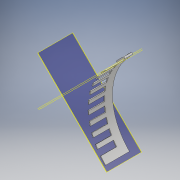
# Autodesk Inventor part: QuarterCircle
Saved by Autodesk Inventor 2018.3 (Build 223284000, 284)
## iProperties
Created: 2021-04-14
Part Number: QuarterCircle
Material: Generic
Document SubType Name: Modeling
Designer: swarmArena
Density: 1 g/cm^3
Appearance: Default
Author: swarmArena
Autodesk Inventor part; units mm, degrees
ref_plane "YZ Plane" through (0, 0, 0) normal (1, 0, 0) x (0, 1, 0)
ref_plane "XZ Plane" through (0, 0, 0) normal (0, 1, 0) x (-1, 0, 0)
ref_plane "XY Plane" through (0, 0, 0) normal (0, 0, 1) x (1, 0, 0)
sketch "Sketch1" plane through (0, 0, 0) normal (0, 1, 0) x (-1, 0, 0)
  circle A0 centre (0, 0) radius 111
  dimension "d13" = 222
  constraints: 1 centre point
  measures "d13" diameter of A0
extrude "Extrusion1" add sketch "Sketch1" along normal blind 45
sketch "Sketch2" plane through (0, 0, 0) normal (0, 1, 0) x (-1, 0, 0)
  circle A0 centre (0, 0) radius 109.5
  dimension "d16" = 219
  constraints: 1 centre point, 1 coincident
  measures "d16" diameter of A0
extrude "Extrusion2" cut sketch "Sketch2" along normal blind 50
sketch "Sketch3" plane through (0, 0, 0) normal (0, 1, 0) x (-1, 0, 0)
  line L0 (0, 0) -> (106.066, 106.066)
  line L1 (106.066, 106.066) -> (0, 212.132)
  line L2 (0, 212.132) -> (-106.066, 106.066)
  line L3 (-106.066, 106.066) -> (0, 0)
  line L4 (0, 0) -> (-106.066, -106.066)
  line L5 (-106.066, -106.066) -> (-212.132, 0)
  line L6 (-212.132, 0) -> (-106.066, 106.066)
  line L7 (-106.066, 106.066) -> (0, 0)
  line L8 (0, 0) -> (-106.066, -106.066)
  line L9 (-106.066, -106.066) -> (0, -212.132)
  line L10 (0, -212.132) -> (106.066, -106.066)
  line L11 (106.066, -106.066) -> (0, 0)
  dimension "d19" = 150
  dimension "d20" = 150
  dimension "d21" = 150
  dimension "d22" = 150
  dimension "d23" = 150
  dimension "d24" = 150
  constraints: 24 end point, 6 parallel, 3 perpendicular
  measures "d19" distance of L2.end L1.end
  measures "d20" distance of L1.end L0.end
  measures "d21" distance of L5.end L6.end
  measures "d22" distance of L4.end L5.end
  measures "d23" distance of L10.end L9.end
  measures "d24" distance of L9.end L8.end
extrude "Extrusion3" cut sketch "Sketch3" along normal blind 60
sketch "Sketch4" plane through (0, 0, 0) normal (1, 0, 0) x (0, 1, 0)
  line L0 (0, -77.4282) -> (0, 77.4282) projected
  line L1 (0, -4) -> (30, -4)
  line L2 (30, -4) -> (30, 6)
  line L3 (30, 6) -> (0, 6)
  line L4 (0, 6) -> (0, -4)
  line L5 (-32.9413, -3) -> (-32.9413, -15.7313) construction
  line L6 (-32.9413, -20) -> (-32.9413, -32.7313) construction
  line L7 (0, -21) -> (30, -21)
  line L8 (30, -11) -> (0, -11)
  line L9 (30, -21) -> (30, -11)
  line L10 (0, -11) -> (0, -21)
  line L11 (-32.9413, -37) -> (-32.9413, -49.7313) construction
  line L12 (0, -38) -> (30, -38)
  line L13 (30, -28) -> (0, -28)
  line L14 (30, -38) -> (30, -28)
  line L15 (0, -28) -> (0, -38)
  line L16 (-32.9413, -54) -> (-32.9413, -66.7313) construction
  line L17 (0, -55) -> (30, -55)
  line L18 (30, -45) -> (0, -45)
  line L19 (30, -55) -> (30, -45)
  line L20 (0, -45) -> (0, -55)
  line L21 (-32.9413, -71) -> (-32.9413, -83.7313) construction
  line L22 (0, -72) -> (30, -72)
  line L23 (30, -62) -> (0, -62)
  line L24 (30, -72) -> (30, -62)
  line L25 (0, -62) -> (0, -72)
  line L26 (0, 23) -> (0, 13)
  line L27 (0, 13) -> (30, 13)
  line L28 (30, 23) -> (0, 23)
  line L29 (30, 13) -> (30, 23)
  line L30 (0, 40) -> (0, 30)
  line L31 (0, 30) -> (30, 30)
  line L32 (30, 40) -> (0, 40)
  line L33 (30, 30) -> (30, 40)
  line L34 (0, 57) -> (0, 47)
  line L35 (0, 47) -> (30, 47)
  line L36 (30, 57) -> (0, 57)
  line L37 (30, 47) -> (30, 57)
  line L38 (0, 74) -> (0, 64)
  line L39 (0, 64) -> (30, 64)
  line L40 (30, 74) -> (0, 74)
  line L41 (30, 64) -> (30, 74)
  line L42 (45, -78.4889) -> (45, 78.4889) projected
  line L43 (45, 0) -> (72.0393, 0)
  point P0 (0, 0)
  point P1 (0, -17)
  point P2 (0, -34)
  point P3 (0, -51)
  point P4 (0, -68)
  point P5 (0, 17)
  point P6 (0, 34)
  point P7 (0, 51)
  point P8 (0, 68)
  dimension "d27" = 30
  dimension "d28" = 10
  dimension "d31" = 17
  dimension "d38" = 17
  dimension "d45" = 6
  constraints: 84 end point, 3 vertical, 2 horizontal, 2 parallel, 1 collinear, 1 midpoint, 1 perpendicular, 1 point on line, 83 other
  measures "d27" distance of L3.end L2.end
  measures "d28" distance of L2.end L1.end
  measures "d31" distance of L5.start L6.start
  measures "d38" distance of point (0, 0) point (0, 17)
  measures "d45" distance between parallel lines of L43 L3
emboss "Emboss1" sketch "Sketch4" operation cut depth 10 direction (1, 0, 0) wrap yes faces at (-80.7319, 30, -73.9771)
ref_plane "Work Plane1" through (-78.4889, 0, 78.4889) normal (-0.7071068, 0, 0.7071068) x (0, -1, 0)
ref_plane "Work Plane2" through (-78.4889, 0, -78.4889) normal (-0.7071068, 0, -0.7071068) x (0, -1, 0)
sketch "Sketch5" plane through (-78.4889, 0, 78.4889) normal (-0.7071068, 0, 0.7071068) x (0, -1, 0)
  line L0 (-30, -10) -> (-45, -10)
  line L1 (-45, -10) -> (-45, 10)
  line L2 (-45, 10) -> (-30, 10)
  line L3 (-30, 10) -> (-30, -10)
  point P0 (0, 0)
  dimension "d46" = 15
  dimension "d47" = 20
  constraints: 8 end point, 2 parallel, 1 horizontal, 1 perpendicular
  measures "d46" distance of L1.end L2.end
  measures "d47" distance of L0.end L1.end
emboss "Emboss2" sketch "Sketch5" operation add depth 3 direction (0.7071068, 0, -0.7071068) wrap yes faces at (-82.8201, 25, -73.9042)
sketch "Sketch7" plane through (-78.4889, 0, 78.4889) normal (-0.7071068, 0, 0.7071068) x (0, -1, 0)
  line L0 (-65, 8) -> (-50, 8)
  line L1 (-50, 8) -> (-50, 2)
  line L2 (-50, 2) -> (-65, 2)
  line L3 (-65, 2) -> (-65, 8)
  point P0 (0, 0)
  dimension "d50" = 15
  dimension "d51" = 6
  constraints: 8 end point, 2 parallel, 1 horizontal, 1 perpendicular
  measures "d50" distance of L1.end L2.end
  measures "d51" distance of L0.end L1.end
emboss "Emboss3" [suppressed]
sketch "Sketch11" plane through (-78.4889, 0, -78.4889) normal (-0.7071068, 0, -0.7071068) x (0, -1, 0)
  line L0 (-50, 3.5) -> (-60, 3.5)
  line L1 (-60, 3.5) -> (-60, 6.5)
  line L2 (-60, 6.5) -> (-50, 6.5)
  line L3 (-50, 6.5) -> (-50, 3.5)
  point P0 (0, 0)
  dimension "d61" = 10
  dimension "d62" = 3
  constraints: 8 end point, 2 parallel, 1 horizontal, 1 perpendicular
  measures "d61" distance of L1.end L2.end
  measures "d62" distance of L0.end L1.end
emboss "Emboss4" [suppressed]
ref_plane "Work Plane3" through (-79.196, 0, -79.196) normal (-0.7071068, 0, -0.7071068) x (0, -1, 0)
sketch "Sketch12" plane through (-79.196, 0, -79.196) normal (-0.7071068, 0, -0.7071068) x (0, -1, 0)
  line L0 (-50, 2) -> (-60, 2)
  line L1 (-60, 2) -> (-60, 8)
  line L2 (-60, 8) -> (-50, 8)
  line L3 (-50, 8) -> (-50, 2)
  point P0 (0, 0)
  dimension "d66" = 10
  dimension "d67" = 6
  constraints: 8 end point, 2 parallel, 1 horizontal, 1 perpendicular
  measures "d66" distance of L1.end L2.end
  measures "d67" distance of L0.end L1.end
emboss "Emboss5" [suppressed]
ref_plane "Work Plane4" through (-77.0746, 0, 77.0746) normal (-0.7071068, 0, 0.7071068) x (0, -1, 0)
sketch "Sketch15" plane through (-77.0746, 0, 77.0746) normal (-0.7071068, 0, 0.7071068) x (0, -1, 0)
  line L0 (-60, 2) -> (-50, 2)
  line L1 (-50, 2) -> (-50, 8)
  line L2 (-50, 8) -> (-60, 8)
  line L3 (-60, 8) -> (-60, 2)
  point P0 (0, 0)
  dimension "d75" = 10
  dimension "d76" = 6
  constraints: 8 end point, 2 parallel, 1 horizontal, 1 perpendicular
  measures "d75" distance of L2.end L1.end
  measures "d76" distance of L1.end L0.end
emboss "Emboss7" [suppressed]
sketch "Sketch16" plane through (-97.9036, 50, 100.7727) normal (0.7172436, 0, 0.6968225) x (0.6968225, 0, -0.7172436)
  line L0 (2.0144, 10) -> (2, 10) projected
  line L1 (0, 0) -> (2, 0) projected
  line L2 (2, 10) -> (1, 10)
  line L3 (1, 10) -> (1, 0)
  line L4 (1, 0) -> (2, 0)
  line L5 (2, 0) -> (2, 10)
  point P0 (140.5, -50)
  constraints: 8 end point, 2 parallel, 1 horizontal, 1 midpoint, 1 perpendicular
sketch "Sketch17" plane through (-93.4475, 50, 104.9182) normal (-0.7467485, 0, -0.6651065) x (-0.6651065, 0, 0.7467485)
  line L0 (-2, 0) -> (-2, 10) projected
  line L1 (-2, 10) -> (0, 10) projected
  line L2 (-2, 0) -> (-1, 0)
  line L3 (-1, 0) -> (-1, 10)
  line L4 (-1, 10) -> (-2, 10)
  line L5 (-2, 10) -> (-2, 0)
  point P0 (-140.5, -50)
  constraints: 8 end point, 2 parallel, 1 horizontal, 1 midpoint, 1 perpendicular
extrude "Extrusion7" [suppressed]
extrude "Extrusion8" [suppressed]
body "Solid1"
